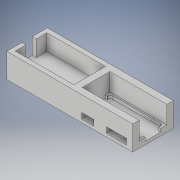
# Autodesk Inventor part: PiHolder
Saved by Autodesk Inventor 2019 (Build 230136000, 136)
## iProperties
Created: 2019-04-12
Part Number: PiHolder
Material: Generic
Document SubType Name: Modeling
Designer: Epsilon
Density: 1 g/cm^3
Appearance: Default
Author: Epsilon
Autodesk Inventor part; units mm, degrees
ref_plane "YZ Plane" through (0, 0, 0) normal (1, 0, 0) x (0, 1, 0)
ref_plane "XZ Plane" through (0, 0, 0) normal (0, 1, 0) x (-1, 0, 0)
ref_plane "XY Plane" through (0, 0, 0) normal (0, 0, 1) x (1, 0, 0)
sketch "Sketch2" plane through (0, 0, 0) normal (0, 1, 0) x (-1, 0, 0)
  line L0 (0, 0) -> (155, 0)
  line L1 (155, 0) -> (155, -50)
  line L2 (155, -50) -> (0, -50)
  line L3 (0, -50) -> (0, 0)
  dimension "d4" = 155
  dimension "d5" = 50
  constraints: 8 end point, 2 parallel, 1 horizontal, 1 perpendicular
  measures "d4" distance of L1.end L2.end
  measures "d5" distance of L0.end L1.end
extrude "Extrusion2" add sketch "Sketch2" along normal blind 30
sketch "Sketch4" plane through (0, 30, 0) normal (0, 1, 0) x (1, 0, 0)
  line L0 (0, 0) -> (0, 50) projected
  line L1 (0, 8) -> (-70, 8)
  line L2 (-70, 8) -> (-70, 42)
  line L3 (-70, 42) -> (0, 42)
  line L4 (0, 42) -> (0, 8)
  line L5 (-155, 50) -> (-155, 0) construction
  line L6 (-155, 25) -> (0, 25) construction
  dimension "d8" = 70
  dimension "d9" = 34
  constraints: 10 end point, 2 midpoint, 2 parallel, 2 perpendicular, 1 horizontal, 1 point on line, 1 other
  measures "d8" distance of L2.end L3.end
  measures "d9" distance of L1.end L2.end
extrude "Extrusion3" cut sketch "Sketch4" against normal blind 26
sketch "Sketch5" plane through (0, 4, 0) normal (0, 1, 0) x (1, 0, 0)
  line L0 (0, 8) -> (-70, 8) projected
  line L1 (-70, 42) -> (0, 42) projected
  line L2 (0, 8) -> (-70, 8)
  line L3 (-70, 8) -> (-70, 21)
  line L4 (-70, 42) -> (0, 42)
  line L5 (0, 42) -> (0, 15.475)
  line L6 (-2.5, 10) -> (-67.5, 10)
  line L7 (-67.5, 10) -> (-67.5, 21)
  line L8 (-67.5, 40) -> (-2.5, 40)
  line L9 (-2.5, 40) -> (-2.5, 34.525)
  line L10 (0, 50) -> (0, 0) construction
  line L11 (0, 25) -> (-70, 25) construction
  line L12 (-70, 8) -> (-70, 42) construction
  line L13 (-35, 8) -> (-35, 40) construction
  line L14 (0, 42) -> (0, 8) projected
  line L15 (-2.5, 15.475) -> (0, 15.475)
  line L16 (0, 34.525) -> (-2.5, 34.525)
  line L17 (-2.5, 15.475) -> (-2.5, 10)
  line L18 (0, 15.475) -> (0, 8)
  line L19 (-70, 8) -> (-70, 42) projected
  line L20 (-67.5, 36) -> (-70, 36)
  line L21 (-70, 36) -> (-70, 21) construction
  line L22 (-70, 21) -> (-67.5, 21)
  line L23 (-67.5, 21) -> (-67.5, 25) construction
  line L24 (-67.5, 36) -> (-67.5, 40)
  line L25 (-67.5, 21) -> (-67.5, 36) construction
  line L26 (-70, 21) -> (-70, 36)
  line L27 (-70, 36) -> (-70, 42)
  dimension "d12" = 65
  dimension "d13" = 30
  dimension "d17" = 19.05
  dimension "d43" = 15
  dimension "d44" = 4
  constraints: 44 end point, 17 parallel, 8 perpendicular, 4 horizontal, 4 midpoint, 3 point on line, 4 other
  measures "d12" distance of L8.start L8.end
  measures "d13" distance of L6.end L8.start
  measures "d17" distance of L16.start L5.end
  measures "d43" distance of L3.end L20.end
  measures "d44" distance between parallel lines of L8 L20
extrude "Extrusion5" add sketch "Sketch5" along normal blind 4 contours L0 L3 L22 L7 L6 L17 L15 L14 | L16 L9 L8 L24 L20 L19 L1 L5
fillet "Fillet2" radius 3 4 edges at (-2.5, 6, -10) (-67.5, 6, -10) (-67.5, 6, -40) (-2.5, 6, -40)
sketch "Sketch7" plane through (-155, 0, 0) normal (0, 0, 1) x (1, 0, 0)
  line L0 (92.4, 4) -> (107.4, 4)
  line L1 (107.4, 4) -> (107.4, 11)
  line L2 (107.4, 11) -> (92.4, 11)
  line L3 (92.4, 11) -> (92.4, 4)
  line L4 (92.4, 7.5) -> (107.4, 7.5) construction
  line L5 (99.9, 11) -> (99.9, 4) construction
  line L6 (90.5, 8) -> (90.5, 4) construction
  line L7 (90.5, 4) -> (149.5, 4) construction
  line L8 (87.5, 4) -> (87.5, 8) projected
  line L9 (122.9, 4) -> (134.9, 4)
  line L10 (134.9, 4) -> (134.9, 11) construction
  line L11 (134.9, 11) -> (122.9, 11)
  line L12 (122.9, 11) -> (122.9, 4)
  line L13 (135.5, 4) -> (147.5, 4)
  line L14 (147.5, 4) -> (147.5, 11)
  line L15 (147.5, 11) -> (135.5, 11)
  line L16 (135.5, 11) -> (135.5, 4) construction
  line L17 (128.9, 11) -> (128.9, 4) construction
  line L18 (141.5, 11) -> (141.5, 4) construction
  line L19 (134.9, 11) -> (135.5, 11) construction
  line L20 (134.9, 11) -> (135.5, 11)
  line L21 (134.9, 4) -> (135.5, 4)
  point P0 (155, 0)
  dimension "d29" = 15
  dimension "d30" = 7
  dimension "d32" = 0
  dimension "d35" = 12.4
  dimension "d36" = 12
  dimension "d37" = 7
  dimension "d38" = 12
  dimension "d39" = 7
  dimension "d40" = 41.4
  dimension "d41" = 54
  constraints: 38 end point, 8 midpoint, 6 parallel, 3 horizontal, 3 perpendicular, 2 point on line, 1 collinear
  measures "d29" distance of L2.end L1.end
  measures "d30" distance of L1.end L0.end
  measures "d32" distance between parallel lines of L7 L0
  measures "d35" distance between parallel lines of L8 L5
  measures "d36" distance of L11.end L10.end
  measures "d37" distance of L10.end L9.end
  measures "d38" distance of L15.end L14.end
  measures "d39" distance of L14.end L13.end
  measures "d40" distance between parallel lines of L8 L17
  measures "d41" distance between parallel lines of L8 L18
extrude "Extrusion7" cut sketch "Sketch7" against normal up to next
sketch "Sketch9" plane through (0, 30, 0) normal (0, 1, 0) x (1, 0, 0)
  line L0 (-78, 44.5) -> (-150, 44.5)
  line L1 (-150, 44.5) -> (-150, 31.35)
  line L2 (-150, 5.5) -> (-78, 5.5)
  line L3 (-78, 5.5) -> (-78, 44.5)
  line L4 (0, 50) -> (0, 0) construction
  line L5 (0, 25) -> (-155, 25) construction
  line L6 (-155, 0) -> (-155, 50) construction
  line L7 (-150, 25) -> (-78, 25) construction
  line L8 (-155, 50) -> (-155, 0) projected
  line L9 (-150, 18.65) -> (-155, 18.65)
  line L10 (-155, 18.65) -> (-155, 31.35)
  line L11 (-155, 31.35) -> (-150, 31.35)
  line L12 (-150, 31.35) -> (-150, 25) construction
  line L13 (-150, 25) -> (-155, 25) construction
  line L14 (-150, 31.35) -> (-150, 25) construction
  line L15 (-150, 18.65) -> (-150, 5.5)
  line L16 (-150, 25) -> (-150, 18.65) construction
  line L17 (-150, 25) -> (-150, 18.65) construction
  dimension "d45" = 72
  dimension "d46" = 39
  dimension "d47" = 5
  dimension "d50" = 12.7
  constraints: 30 end point, 8 parallel, 5 perpendicular, 4 midpoint, 2 collinear, 2 horizontal, 2 point on line
  measures "d45" distance between parallel lines of L3 L1
  measures "d46" distance between parallel lines of L2 L0
  measures "d47" distance between parallel lines of L6 L1
  measures "d50" distance between parallel lines of L9 L11
extrude "Extrusion8" cut sketch "Sketch9" against normal blind 20
equation "\"d37\" = d30"
equation "\"d38\" = d36"
equation "\"d39\" = d37"
body "Solid2"
